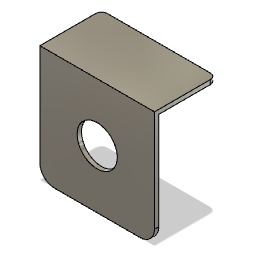
Motor clamp v2 (Autodesk Fusion 360 design; units mm, degrees)
Autodesk Fusion 360 part; units mm, degrees
note: some values were not read from the file. Set by a fixed rule: which sketch regions a step uses.
sketch "Sketch1" plane through (0, 0, 0) normal (0, 1, 0) x (1, 0, 0)
  line L0 (18, 10.75) -> (-18, 10.75)
  line L1 (-20, 8.75) -> (-20, -10.75)
  line L2 (-20, -10.75) -> (20, -10.75)
  line L3 (20, -10.75) -> (20, 8.75)
  line L4 (20, 10.75) -> (-20, -10.75) construction
  line L5 (-20, 10.75) -> (20, -10.75) construction
  arc A0 (-18, 10.75) -> (-20, 8.75) centre (-18, 8.75) ccw
  arc A1 (20, 8.75) -> (18, 10.75) centre (18, 8.75) ccw
  dimension "d1" = 40
  dimension "d2" = 21.5
  dimension "d3" = 2
  constraint horizontal L0
  constraint perpendicular L0 L1
  constraint parallel L0 L2
  constraint parallel L1 L3
  constraint coincident L4 origin
  constraint coincident L5 origin
  constraint coincident L5.start L0
  constraint coincident L5.start L1
  constraint tangent L0 A0
  constraint tangent L1 A0
  constraint coincident L4.start L0
  constraint coincident L4.start L3
  constraint tangent L0 A1
  constraint tangent L3 A1
  constraint equal A0 A1
  measures "d1" distance of L1.end L2.end
  measures "d2" distance of L5.start L1.end
  measures "d3" radius of A0
extrude "Extrude1" add sketch "Sketch1" along normal blind 1.5
sketch "Sketch2" plane through (0, 0, 10.75) normal (0, 0, 1) x (1, 0, 0)
  line L0 (-20, 0) -> (20, 0)
  line L1 (20, 0) -> (20, 1.5)
  line L2 (20, 1.5) -> (-20, 1.5)
  line L3 (-20, 1.5) -> (-20, 0)
  line L4 (-20, 1.5) -> (20, 1.5)
  line L5 (20, 1.5) -> (20, -34)
  line L6 (15, -39) -> (-15, -39)
  line L7 (-20, -34) -> (-20, 1.5)
  circle A0 centre (0, -18.75) radius 7
  arc A1 (-20, -34) -> (-15, -39) centre (-15, -34) ccw
  arc A2 (15, -39) -> (20, -34) centre (15, -34) ccw
  point P0 (-20, -39)
  dimension "d7" = 40.5
  dimension "d8" = 14
  dimension "d11" = 5
  constraint horizontal L4
  constraint vertical L5
  constraint horizontal L6
  constraint vertical L7
  constraint coincident L2.end L3.start
  constraint coincident P0 L7
  constraint coincident P0 L6
  constraint tangent L7 A1
  constraint tangent L6 A1
  constraint tangent L5 A2
  constraint tangent L6 A2
  constraint equal A1 A2
  measures "d7" distance of L2.end P0
  measures "d8" diameter of A0
  measures "d11" radius of A1
extrude "Extrude2" add sketch "Sketch2" against normal blind 1.5
